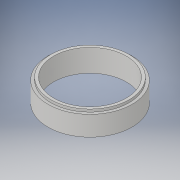
# Autodesk Inventor part: Aluminum Retainer 8-inch v1
Saved by Autodesk Inventor 2017 (Build 210142000, 142)
## iProperties
Created: 2016-07-07
Part Number: Aluminum Retainer 8-inch v1
Material: Generic
Document SubType Name: Modeling
Designer: Bill
Density: 1 g/cm^3
Appearance: Default
Author: Bill
Autodesk Inventor part; units mm, degrees
ref_plane "YZ Plane" through (0, 0, 0) normal (1, 0, 0) x (0, 1, 0)
ref_plane "XZ Plane" through (0, 0, 0) normal (0, 1, 0) x (-1, 0, 0)
ref_plane "XY Plane" through (0, 0, 0) normal (0, 0, 1) x (1, 0, 0)
sketch "Sketch1" plane through (0, 0, 0) normal (0, 0, 1) x (1, 0, 0)
  line L0 (-82.5669, 28.2647) -> (-88.9169, 28.2647)
  line L1 (-88.9169, 28.2647) -> (-88.9169, 22.3211)
  line L2 (-88.9169, 22.3211) -> (-95.2669, 22.3211)
  line L3 (-95.2669, 22.3211) -> (-95.2669, -22.5353)
  line L4 (-95.2669, -22.5353) -> (-82.5669, -22.5353)
  line L5 (-82.5669, -22.5353) -> (-82.5669, 28.2647)
  line L6 (0, -32.6953) -> (0, 38.4247) projected
  point P0 (0, 0)
  dimension "d0" = 50.8
  dimension "d1" = 6.35
  dimension "d2" = 6.35
  dimension "d3" = 5.9436
  dimension "d4" = 95.2669
  constraints: 12 end point, 5 perpendicular, 1 horizontal
  measures "d0" distance between parallel lines of L4 L0
  measures "d1" distance of L1.end L2.end
  measures "d2" distance of L0.start L0.end
  measures "d3" distance of L0.end L1.end
  measures "d4" distance from line of point (0, 0) L3
revolve "Revolution1" add sketch "Sketch1" angle 360 about axis through (0, -10, 0) along (0, 1, 0)
body "Solid1"
